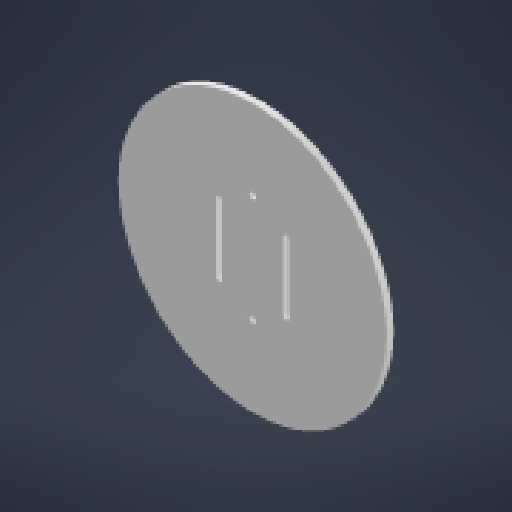
# Autodesk Inventor part: TableStandMiddle
Saved by Autodesk Inventor 2026.3 (Build 303398000, 398)
## iProperties
Created: 2026-06-26
Part Number: TableStandMiddle
Material: Generic
Document SubType Name: Modeling
Designer: frede
Density: 1 g/cm^3
Appearance: Default
Author: frede
Autodesk Inventor part; units mm, degrees
ref_plane "YZ Plane" through (0, 0, 0) normal (1, 0, 0) x (0, 1, 0)
ref_plane "XZ Plane" through (0, 0, 0) normal (0, 1, 0) x (-1, 0, 0)
ref_plane "XY Plane" through (0, 0, 0) normal (0, 0, 1) x (1, 0, 0)
sketch "Sketch1" plane through (0, 0, 0) normal (0, 0, 1) x (1, 0, 0)
  circle A0 centre (0, 0) radius 100
  arc A1 (-22.8, 25) -> (-27.2, 25) centre (-25, 25) ccw
  arc A2 (-27.2, -25) -> (-22.8, -25) centre (-25, -25) ccw
  line L0 (-27.2, 25) -> (-27.2, -25)
  line L1 (-22.8, 25) -> (-22.8, -25)
  arc A3 (22.8, -25) -> (27.2, -25) centre (25, -25) ccw
  arc A4 (27.2, 25) -> (22.8, 25) centre (25, 25) ccw
  line L2 (27.2, -25) -> (27.2, 25)
  line L3 (22.8, -25) -> (22.8, 25)
  line L4 (-25, 25) -> (-25, -25)
  dimension "d0" = 200
  dimension "d1" = 4.4
  dimension "d2" = 4.4
  dimension "d3" = 50
  dimension "d4" = 25
  dimension "d7" = 360
  dimension "d9" = 25
  constraints: 10 end point, 8 point on circle, 5 centre point, 2 tangent, 1 coincident, 1 vertical, 21 other
  measures "d0" diameter of A0
  measures "d1" diameter of A1
  measures "d2" diameter of A2
  measures "d3" distance of L4.end L4.start
  measures "d4" horizontal distance of point (0, 0) L4.start
  measures "d9" distance from line of L4 point (0, 0)
extrude "Extrusion1" add sketch "Sketch1" along normal blind 5
fillet "Fillet1" radius 0.25 18 edges at (-100, 0, 5) (-100, 0, 0) (25, -27.2, 5) (22.8, 0, 5) (25, 27.2, 5) (27.2, 0, 5) (25, 27.2, 0) (27.2, 0, 0) (25, -27.2, 0) (22.8, 0, 0) (-25, -27.2, 5) (-27.2, 0, 5) (-25, 27.2, 5) (-22.8, 0, 5) (-25, -27.2, 0) (-27.2, 0, 0) (-25, 27.2, 0) (-22.8, 0, 0)
sketch "Sketch2" plane through (0, 0, 0) normal (0, 0, -1) x (-1, 0, 0)
  circle A0 centre (0, 40) radius 2.2
  circle A1 centre (0, -40) radius 2.2
  point P0 (0, 0)
  dimension "d13" = 4.4
  dimension "d14" = 4.4
  dimension "d15" = 80
  dimension "d16" = 40
  constraints: 2 centre point
  measures "d13" diameter of A0
  measures "d14" diameter of A1
  measures "d15" distance of A1.centre A0.centre
  measures "d16" distance of point (0, 0) A1.centre
extrude "Extrusion2" cut sketch "Sketch2" against normal up to surface (5 mm away)
sketch "Sketch3" plane through (0, 0, 0) normal (0, 0, -1) x (-1, 0, 0)
  circle A0 centre (0, 40) radius 2.2 projected
  line L0 (-2.0785, 36.4) -> (-4.1569, 40)
  line L1 (-4.1569, 40) -> (-2.0785, 43.6)
  line L2 (-2.0785, 43.6) -> (2.0785, 43.6)
  line L3 (2.0785, 43.6) -> (4.1569, 40)
  line L4 (4.1569, 40) -> (2.0785, 36.4)
  line L5 (2.0785, 36.4) -> (-2.0785, 36.4)
  circle A1 centre (0, -40) radius 2.2 projected
  line L6 (2.0785, -36.4) -> (4.1569, -40)
  line L7 (4.1569, -40) -> (2.0785, -43.6)
  line L8 (2.0785, -43.6) -> (-2.0785, -43.6)
  line L9 (-2.0785, -43.6) -> (-4.1569, -40)
  line L10 (-4.1569, -40) -> (-2.0785, -36.4)
  line L11 (-2.0785, -36.4) -> (2.0785, -36.4)
  point P0 (0, 0)
  dimension "d19" = 7.2
  dimension "d20" = 7.2
  constraints: 24 end point, 2 coincident, 26 other
  measures "d19" distance between parallel lines of L5 L2
  measures "d20" distance between parallel lines of L8 L11
extrude "Extrusion3" cut sketch "Sketch3" against normal blind 3.2
fillet "Fillet2" radius 0.25 28 edges at (-3.1177, -38.2, 0) (0, -36.4, 0) (3.1177, -38.2, 0) (3.1177, -41.8, 0) (0, -43.6, 0) (-3.1177, -41.8, 0) (2.2, -40, 3.2) (-3.1177, -38.2, 3.2) (2.2, -40, 5) (0, -36.4, 3.2) (3.1177, -38.2, 3.2) (3.1177, -41.8, 3.2) (0, -43.6, 3.2) (-3.1177, -41.8, 3.2) (-3.1177, 41.8, 0) (-3.1177, 38.2, 0) (0, 43.6, 0) (3.1177, 41.8, 0) (3.1177, 38.2, 0) (0, 36.4, 0) (2.2, 40, 3.2) (2.2, 40, 5) (-3.1177, 41.8, 3.2) (0, 43.6, 3.2) (3.1177, 41.8, 3.2) (3.1177, 38.2, 3.2) (0, 36.4, 3.2) (-3.1177, 38.2, 3.2)
equation "\"d2\" = d1"
equation "\"d4\" = 0.5 * d3"
body "Solid1"
